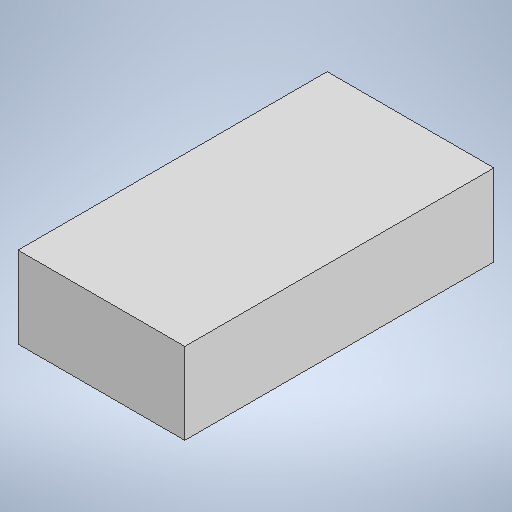
# Autodesk Inventor part: Battery_Holder
Saved by Autodesk Inventor 2025 (Build 290162000, 162)
## iProperties
Created: 2025-10-15
Part Number: Battery_Holder
Material: Типовые
Document SubType Name: Modeling
Designer: Admin
Density: 1 g/cm^3
Appearance: По умолчанию
Author: Admin
Autodesk Inventor part; units mm, degrees
ref_plane "YZ Plane" through (0, 0, 0) normal (1, 0, 0) x (0, 1, 0)
ref_plane "XZ Plane" through (0, 0, 0) normal (0, 1, 0) x (-1, 0, 0)
ref_plane "XY Plane" through (0, 0, 0) normal (0, 0, 1) x (1, 0, 0)
sketch "Эскиз1" plane through (0, 0, 0) normal (0, 1, 0) x (-1, 0, 0)
  line L0 (0, 0) -> (41, 0)
  line L1 (41, 0) -> (41, -76)
  line L2 (41, -76) -> (0, -76)
  line L3 (0, -76) -> (0, 0)
  line L4 (38.493, -5.6262) -> (20.493, -5.6262)
  line L5 (20.493, -5.6262) -> (20.493, -70.6262)
  line L6 (20.493, -70.6262) -> (38.493, -70.6262)
  line L7 (38.493, -70.6262) -> (38.493, -5.6262)
  line L8 (18.991, -5.4252) -> (0.991, -5.4252)
  line L9 (0.991, -5.4252) -> (0.991, -70.4252)
  line L10 (0.991, -70.4252) -> (18.991, -70.4252)
  line L11 (18.991, -70.4252) -> (18.991, -5.4252)
  dimension "d0" = 41
  dimension "d1" = 76
  dimension "d2" = 18
  dimension "d3" = 65
  dimension "d4" = 18
  dimension "d5" = 65
  constraints: 24 end point, 6 parallel, 3 horizontal, 3 perpendicular
  measures "d0" distance of L1.end L2.end
  measures "d1" distance of L2.end L0.start
  measures "d2" distance of L6.end L5.end
  measures "d3" distance of L6.end L4.start
  measures "d4" distance of L10.end L9.end
  measures "d5" distance of L10.end L8.start
extrude "Выдавливание1" add sketch "Эскиз1" along normal blind 20 contours L0 L1 L2 L3 | L7 L6 L5 L4 | L11 L10 L9 L8
extrude "Выдавливание2" cut sketch "Эскиз1" along normal blind 18 contours L7 L6 L5 L4 | L11 L10 L9 L8
